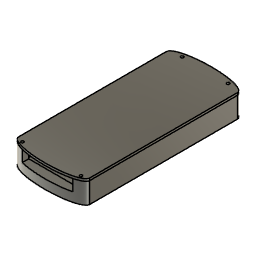
ESP32S3 (Autodesk Fusion 360 design; units mm, degrees)
Autodesk Fusion 360 part; units mm, degrees
sketch "Boceto1" plane through (0, 0, 0) normal (0, 0, 1) x (1, 0, 0)
  line L0 (14.5, -32.25) -> (-14.5, -32.25)
  line L1 (-14.5, -32.25) -> (-14.5, 32.25)
  line L2 (-14.5, 32.25) -> (14.5, 32.25)
  line L3 (14.5, 32.25) -> (14.5, -32.25)
  line L4 (14.5, -32.25) -> (-14.5, 32.25) construction
  line L5 (-14.5, -32.25) -> (14.5, 32.25) construction
  line L6 (-15.5, 32.25) -> (-15.5, -32.25)
  line L7 (15.5, -32.25) -> (15.5, 32.25)
  ellipse E0 centre (0, -32.25) end of major axis (15.5, -32.25) minor radius 4 (-15.5, -32.25) -> (15.5, -32.25) ccw
  line L8 (-14.5, -31.1048) -> (-15.3184, -32.8605) construction
  line L9 (-15.5, 33.25) -> (-14.5, 31.1048) construction
  line L10 (14.5, -31.1048) -> (15.3184, -32.8605) construction
  line L11 (15.3184, 32.8605) -> (14.5, 31.1048) construction
  line L12 (0, 0) -> (-14.3203, -30.7194) construction
  ellipse E1 centre (0, 32.25) end of major axis (15.5, 32.25) minor radius 4 (15.5, 32.25) -> (-15.5, 32.25) ccw
  dimension "d1" = 29
  dimension "d2" = 64.5
  dimension "d5" = 8
  dimension "d6" = 8
  constraint horizontal L0
  constraint perpendicular L0 L1
  constraint parallel L0 L2
  constraint parallel L1 L3
  constraint coincident L4 L12.start
  constraint coincident L5 L12.start
  constraint coincident L12.start origin
  constraint parallel L6 L7
  constraint coincident L12.start L11
  constraint coincident L12.start L9
  constraint midpoint L2 E1.centre
  constraint midpoint L0 E0.centre
  constraint coincident L8.end E0
  constraint coincident L1 L8.start
  constraint collinear L8 L11
  constraint collinear L9 L10
  constraint coincident L3 L10.start
  constraint coincident E0 L10.end
  constraint coincident L11.start E1
  constraint collinear L11 L12
  constraint coincident L3 L11.end
  constraint coincident L1 L9.end
  measures "d1" distance of L1.end L2.end
  measures "d2" distance of L0.end L1.end
extrude "Extruir1" add sketch "Boceto1" against normal blind 1 contours L0 L1 L2 L3 | L6 L7 E0 E1 makes body 1
extrude "Extruir3" add sketch "Boceto1" along normal blind 8 bodies 1
extrude "Extruir4" add sketch "Boceto1" along normal blind 1 from surface at 8 separate body contours L0 L1 L2 L3 | L6 L7 E0 E1 makes body 2
ref_plane "PlanoDeObra1" through (0, -36.25, 0) normal (0, 1, 0) x (0, 0, 1)
sketch "Boceto3" plane through (0, -36.25, 0) normal (0, 1, 0) x (1, 0, 0)
  line L0 (-15.5, -8) -> (-15.5, 1)
  line L1 (15.5, 1) -> (-15.5, 1)
  line L2 (15.5, 1) -> (15.5, -8)
  line L3 (-15.5, -8) -> (15.5, -8)
  line L4 (0, -8) -> (0, -3) construction
  line L5 (0, -3) -> (-11, -3)
  line L6 (0, -3) -> (11, -3)
  line L7 (-11, -3) -> (-11, -8)
  line L8 (11, -3) -> (11, -8)
  line L9 (11, -8) -> (-11, -8)
  dimension "d21" = 5
  dimension "d22" = 11
  dimension "d23" = 11
  constraint midpoint L3 L4.start
  constraint perpendicular L3 L4
  constraint perpendicular L4 L5
  constraint perpendicular L4 L6
  constraint coincident L3 L7.end
  constraint perpendicular L3 L7
  constraint coincident L3 L8.end
  constraint perpendicular L3 L8
  measures "d21" distance of L4.start L4.end
  measures "d22" distance of L4.end L5.end
  measures "d23" distance of L4.end L6.end
extrude "Extruir5" cut sketch "Boceto3" along normal blind 14 contours L3 L5 L6 L7 L8 L9 bodies 1
ref_plane "PlanoDeObra2" through (0, 32.25, 4) normal (0, -1, 0) x (1, 0, 0)
sketch "Boceto4" plane through (0, 32.25, 0) normal (0, -1, 0) x (-1, 0, 0)
  line L0 (14.5, 0) -> (-14.5, 0)
  line L1 (-14.5, 0) -> (-14.5, -8)
  line L2 (-14.5, -8) -> (14.5, -8)
  line L3 (14.5, -8) -> (14.5, 0)
  line L4 (0, -8) -> (0, 0) construction
  line L5 (-6, -2.75) -> (6, -2.75)
  line L6 (6, -2.75) -> (6, -5.25)
  line L7 (6, -5.25) -> (-6, -5.25)
  line L8 (-6, -5.25) -> (-6, -2.75)
  line L9 (-6, -2.75) -> (6, -5.25) construction
  line L10 (6, -2.75) -> (-6, -5.25) construction
  point P0 (0, -4)
  dimension "d27" = 12
  dimension "d28" = 2.5
  constraint midpoint L2 L4.start
  constraint coincident L4.end origin
  constraint horizontal L5
  constraint perpendicular L5 L6
  constraint parallel L5 L7
  constraint parallel L6 L8
  constraint coincident L9 P0
  constraint coincident L10 P0
  constraint midpoint L4 P0
  measures "d27" distance of L6.end L7.end
  measures "d28" distance of L5.end L6.end
extrude "Extruir6" cut sketch "Boceto4" against normal blind 11 contours L5 L6 L7 L8 bodies 1
sketch "Boceto7" plane through (0, 0, 9) normal (0, 0, 1) x (-1, 0, 0)
  ellipse E0 centre (0, -32.25) end of major axis (-15.5, -32.25) minor radius 4 (-15.5, -32.25) -> (15.5, -32.25) ccw
  line L0 (15.5, -32.25) -> (15.5, 32.25)
  ellipse E1 centre (0, 32.25) end of major axis (-15.5, 32.25) minor radius 4 (15.5, 32.25) -> (-15.5, 32.25) ccw
  line L1 (-15.5, 32.25) -> (-15.5, -32.25)
  line L2 (-11, 32.25) -> (11, 32.25)
  line L3 (11, 32.25) -> (11, 35.0681)
  ellipse E2 centre (0, 32.25) end of major axis (-15.5, 32.25) minor radius 4 (11, 35.0681) -> (-11, 35.0681) ccw
  line L4 (-11, 35.0681) -> (-11, 32.25)
  line L5 (14.5, -32.25) -> (14.5, 32.25)
  line L6 (14.5, 32.25) -> (-14.5, 32.25)
  line L7 (-14.5, 32.25) -> (-14.5, -32.25)
  line L8 (-14.5, -32.25) -> (14.5, -32.25)
  line L9 (-14.5, 32.25) -> (-12.75, 32.25) construction
  line L10 (-12.75, 32.25) -> (-12.75, 33.25) construction
  circle A0 centre (-12.75, 33.25) radius 0.6
  line L11 (14.5, 32.25) -> (12.75, 32.25)
  line L12 (12.75, 32.25) -> (12.75, 33.25) construction
  circle A1 centre (12.75, 33.25) radius 0.6
  line L13 (0, -32.25) -> (0, -36.25)
  line L14 (0, -32.25) -> (10, -32.25)
  line L15 (0, -32.25) -> (-10, -32.25)
  line L16 (-10, -32.25) -> (-10, -33.65) construction
  circle A2 centre (-10, -33.65) radius 0.6
  line L17 (10, -32.25) -> (10, -33.65) construction
  circle A3 centre (10, -33.65) radius 0.6
  dimension "d31" = 1.75
  dimension "d32" = 1
  dimension "d33" = 1.2
  dimension "d34" = 1.75
  dimension "d35" = 1
  dimension "d36" = 1.2
  dimension "d37" = 10
  dimension "d38" = 10
  dimension "d39" = 1.4
  dimension "d40" = 1.2
  dimension "d41" = 1.4
  dimension "d42" = 1.2
  constraint coincident L6.end L7.start
  constraint perpendicular L4 L9
  constraint perpendicular L9 L10
  constraint coincident L10.end A0.centre
  constraint coincident L5.end L6.start
  constraint perpendicular L3 L11
  constraint perpendicular L6 L12
  constraint coincident L12.end A1.centre
  constraint coincident E0.centre L13.start
  constraint coincident E0 L13.end
  constraint perpendicular L8 L13
  constraint perpendicular L5 L14
  constraint perpendicular L13 L15
  constraint perpendicular L8 L16
  constraint coincident L16.end A2.centre
  constraint perpendicular L14 L17
  constraint coincident L17.end A3.centre
  measures "d31" distance of L6.end L9.end
  measures "d32" distance of L9.end L10.end
  measures "d33" diameter of A0
  measures "d34" distance of L5.end L11.end
  measures "d35" distance of L11.end L12.end
  measures "d36" diameter of A1
  measures "d37" distance of E0.centre L14.end
  measures "d38" distance of E0.centre L15.end
  measures "d39" distance of L15.end L16.end
  measures "d40" diameter of A2
  measures "d41" distance of L14.end L17.end
  measures "d42" diameter of A3
extrude "Extruir7" cut sketch "Boceto7" against normal blind 8 contours A0 | A1 | A2 | A3 bodies 1 2
sketch "Boceto8" plane through (-15.5, 0, 0) normal (-1, 0, 0) x (0, -1, 0)
  line L0 (-32.25, 8) -> (-32.25, -1)
  line L1 (-32.25, -1) -> (32.25, -1)
  line L2 (32.25, -1) -> (32.25, 8)
  line L3 (32.25, 8) -> (-32.25, 8)
  line L4 (-32.25, 3.5) -> (-29.25, 3.5) construction
  circle A0 centre (-29.25, 3.5) radius 0.9
  line L5 (-29.25, 3.5) -> (-26.75, 3.5) construction
  circle A1 centre (-26.75, 3.5) radius 0.9
  dimension "d45" = 3
  dimension "d46" = 1.8
  dimension "d47" = 2.5
  dimension "d48" = 1.8
  constraint midpoint L0 L4.start
  constraint perpendicular L0 L4
  constraint coincident L4.end A0.centre
  constraint parallel L4 L5
  constraint coincident L5.end A1.centre
  measures "d45" distance of L4.start L4.end
  measures "d46" diameter of A0
  measures "d47" distance of L4.end L5.end
  measures "d48" diameter of A1
extrude "Extruir8" cut sketch "Boceto8" against normal blind 11 contours A0 | A1 bodies 1
sketch "Boceto10" plane through (0, 0, 0) normal (0, 0, 1) x (-1, 0, 0)
  line L0 (14.5, -32.25) -> (14.5, 32.25)
  line L1 (14.5, 32.25) -> (-14.5, 32.25)
  line L2 (-14.5, 32.25) -> (-14.5, -32.25)
  line L3 (-14.5, -32.25) -> (14.5, -32.25)
  line L4 (-9, 13) -> (9, 13) construction
  line L5 (9, 13) -> (9, -13) construction
  line L6 (9, -13) -> (-9, -13) construction
  line L7 (-9, -13) -> (-9, 13) construction
  line L8 (-9, 13) -> (9, -13) construction
  line L9 (9, 13) -> (-9, -13) construction
  line L10 (0, -13) -> (0, -12) construction
  line L11 (0, -12) -> (1.5, -12)
  line L12 (0, -12) -> (-1.5, -12)
  line L13 (1.5, -12) -> (1.5, -1)
  line L14 (-1.5, -12) -> (-1.5, -1)
  line L15 (1.5, -1) -> (-1.5, -1)
  line L16 (-10, 14) -> (10, 14) construction
  line L17 (10, 14) -> (10, -14) construction
  line L18 (10, -14) -> (-10, -14) construction
  line L19 (-10, -14) -> (-10, 14) construction
  line L20 (-10, 14) -> (10, -14) construction
  line L21 (10, 14) -> (-10, -14) construction
  circle A0 centre (0, -14) radius 0.6
  circle A1 centre (0, 14) radius 0.6
  dimension "d56" = 18
  dimension "d57" = 26
  dimension "d58" = 1
  dimension "d59" = 1.5
  dimension "d60" = 1.5
  dimension "d61" = 11
  dimension "d62" = 11
  dimension "d63" = 20
  dimension "d64" = 28
  dimension "d65" = 1.2
  dimension "d66" = 1.2
  constraint horizontal L4
  constraint perpendicular L4 L5
  constraint parallel L4 L6
  constraint parallel L5 L7
  constraint coincident L8 origin
  constraint coincident L9 origin
  constraint midpoint L6 L10.start
  constraint perpendicular L6 L10
  constraint perpendicular L10 L11
  constraint perpendicular L10 L12
  constraint perpendicular L11 L13
  constraint perpendicular L12 L14
  constraint horizontal L16
  constraint perpendicular L16 L17
  constraint parallel L16 L18
  constraint parallel L17 L19
  constraint coincident L20 origin
  constraint coincident L21 origin
  constraint midpoint L18 A0.centre
  constraint midpoint L16 A1.centre
  measures "d56" distance of L5.end L6.end
  measures "d57" distance of L4.end L5.end
  measures "d58" distance of L10.start L10.end
  measures "d59" distance of L10.end L11.end
  measures "d60" distance of L10.end L12.end
  measures "d61" distance of L11.end L13.end
  measures "d62" distance of L12.end L14.end
  measures "d63" distance of L17.end L18.end
  measures "d64" distance of L16.end L17.end
  measures "d65" diameter of A0
  measures "d66" diameter of A1
extrude "Extruir9" cut sketch "Boceto10" against normal blind 4 contours L11 L12 L13 L14 L15 | A0 | A1 bodies 1
equation "d15 = 5 mm + 3 mm"
equation "d31 = ( 3.5 / 2 ) * 1 mm"
equation "d34 = ( 3.5 / 2 ) * 1 mm"
named bodies: "ESP32S3_CAS", "ESP32S3_TAP"
